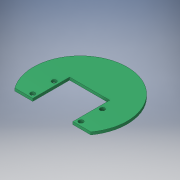
# Autodesk Inventor part: Platine
Saved by Autodesk Inventor 2016 (Build 200138000, 138)
## iProperties
Created: 2016-04-10
Part Number: Platine
Material: Generisch
Document SubType Name: Modeling
Designer: Johann
Density: 1 g/cm^3
Appearance: Glatt - dunkelseegrün
Author: Johann
Autodesk Inventor part; units mm, degrees
ref_plane "YZ Plane" through (0, 0, 0) normal (1, 0, 0) x (0, 1, 0)
ref_plane "XZ Plane" through (0, 0, 0) normal (0, 1, 0) x (-1, 0, 0)
ref_plane "XY Plane" through (0, 0, 0) normal (0, 0, 1) x (1, 0, 0)
sketch "Skizze1" plane through (0, 0, 0) normal (0, 0, 1) x (1, 0, 0)
  line L0 (-15, -20.5) -> (-15, 7)
  line L1 (-15, 7) -> (15, 7)
  line L2 (15, 7) -> (15, -20.5)
  arc A0 (28.3681, -20.5) -> (-28.3681, -20.5) centre (0, 0) ccw
  line L3 (-15, -20.5) -> (-28.3681, -20.5)
  line L4 (15, -20.5) -> (28.3681, -20.5)
  circle A1 centre (-18, -1.5) radius 1.7
  circle A2 centre (18, -1.5) radius 1.7
  circle A3 centre (-18, -17.5) radius 1.7
  circle A4 centre (18, -17.5) radius 1.7
  point P0 (0, 7)
  dimension "d0" = 3.4
  dimension "d5" = 3
  dimension "d6" = 3
  dimension "d7" = 32.6
  dimension "d8" = 35
  dimension "d9" = 16
  dimension "d12" = 3
  dimension "d14" = 20.5
  dimension "d15" = 27.5
  constraints: 10 end point, 5 centre point, 3 equal radius, 3 vertical alignment, 2 horizontal alignment, 2 perpendicular, 2 point on circle, 1 coincident, 1 collinear, 1 horizontal, 1 midpoint, 1 vertical
  measures "d0" diameter of A1
  measures "d5" distance from line of L0 A1.centre
  measures "d6" distance from line of L2 A2.centre
  measures "d8" radius of A0
  measures "d9" distance of A3.centre A1.centre
  measures "d12" distance from line of L4 A4.centre
  measures "d14" distance from line of L3 point (0, 0)
  measures "d15" distance of L0.start L0.end
extrude "Extrusion1" add sketch "Skizze1" along normal blind 2
equation "\"d6\" = d5"
equation "\"d12\" = d5"
